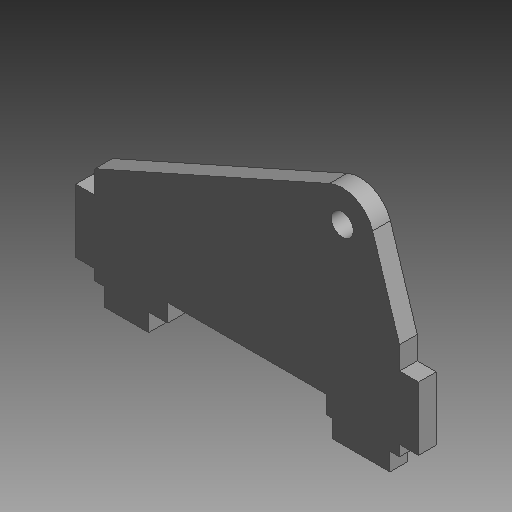
# Autodesk Inventor part: Part15
Saved by Autodesk Inventor 2019.2 (Build 232265000, 265)
## iProperties
Part Number: Part15
Material: Generic
Document SubType Name: Modeling
Designer: richard.girt
Mass: 3.36712 g
Surface Area: 29.1284 cm^2
Volume: 3.36712 cm^3
Density: 1 g/cm^3
Appearance: Default
Author: richard.girt
Autodesk Inventor part; units mm, degrees
note: some values were not read from the file. Chosen so that the rebuilt part matches the saved one: sketch regions of "Extrusion1".
ref_plane "YZ Plane" through (0, 0, 0) normal (1, 0, 0) x (0, 1, 0)
ref_plane "XZ Plane" through (0, 0, 0) normal (0, 1, 0) x (-1, 0, 0)
ref_plane "XY Plane" through (0, 0, 0) normal (0, 0, 1) x (1, 0, 0)
sketch "Sketch1" plane through (0, 0, 0) normal (0, 0, 1) x (1, 0, 0)
  line L0 (24, 7.65) -> (-24, 7.65)
  line L1 (-24, 7.65) -> (-24, -7.65)
  line L2 (-24, -7.65) -> (24, -7.65)
  line L3 (24, -7.65) -> (24, 7.65)
  line L4 (24, 7.65) -> (-24, -7.65) construction
  line L5 (-24, 7.65) -> (24, -7.65) construction
  line L6 (-22.5, -7.65) -> (-15.5, -7.65)
  line L7 (-15.5, -7.65) -> (-15.5, -10.45)
  line L8 (-15.5, -10.45) -> (-22.5, -10.45)
  line L9 (-22.5, -10.45) -> (-22.5, -7.65)
  line L10 (22.5, -7.65) -> (13.5, -7.65)
  line L11 (13.5, -7.65) -> (13.5, -10.45)
  line L12 (13.5, -10.45) -> (22.5, -10.45)
  line L13 (22.5, -10.45) -> (22.5, -7.65)
  line L14 (24, -5.95) -> (27, -5.95)
  line L15 (27, -5.95) -> (27, 4.05)
  line L16 (27, 4.05) -> (24, 4.05)
  line L17 (24, 4.05) -> (24, -5.95)
  line L18 (-24, -5.95) -> (-27, -5.95)
  line L19 (-27, -5.95) -> (-27, 4.05)
  line L20 (-27, 4.05) -> (-24, 4.05)
  line L21 (-24, 4.05) -> (-24, -5.95)
  line L22 (-12.5, -7.65) -> (12.5, -7.65)
  line L23 (12.5, -7.65) -> (12.5, -4.85)
  line L24 (12.5, -4.85) -> (-12.5, -4.85)
  line L25 (-12.5, -4.85) -> (-12.5, -7.65)
  circle A0 centre (15, 19.55) radius 1.75
  arc A1 (19.768, 21.0552) -> (12.9654, 24.1173) centre (15, 19.55) ccw
  line L26 (-24, 7.65) -> (12.9654, 24.1173)
  line L27 (24, 7.65) -> (19.768, 21.0552)
  point P0 (0, 0)
  point P1 (-25.5, -5.95)
  point P2 (25.5, -5.95)
  point P3 (25.5, 4.05)
  point P4 (-25.5, 4.05)
  point P5 (0, -4.85)
  point P6 (0, 0)
  dimension "d0" = 48
  dimension "d1" = 15.3
  dimension "d2" = 3.5
  dimension "d3" = 30
  dimension "d4" = 2.8
  dimension "d5" = 12
  dimension "d6" = 3
  dimension "d7" = 4.5
  dimension "d8" = 10
  dimension "d9" = 25
  dimension "d10" = 7
  dimension "d11" = 9
  dimension "d12" = 4.5
  dimension "d13" = 4.5
  dimension "d14" = 10
  constraints: 56 end point, 12 parallel, 8 midpoint, 6 horizontal, 6 perpendicular, 6 point on line, 2 centre point, 2 equal length, 2 horizontal alignment, 2 point on circle, 2 tangent, 1 coincident, 1 vertical alignment
  measures "d0" distance of L1.end L2.end
  measures "d1" distance of L0.end L1.end
  measures "d2" diameter of A0
  measures "d3" distance from line of L12 A0.centre
  measures "d4" distance of L12.end L10.start
  measures "d5" distance from line of A0.centre L15
  measures "d6" distance of L14.start L14.end
  measures "d7" distance between parallel lines of L14 L12
  measures "d8" distance of L14.end L15.end
  measures "d9" distance of L23.end L24.end
  measures "d10" distance of L7.end L8.end
  measures "d11" distance of L11.end L12.end
  measures "d12" distance between parallel lines of L13 L15
  measures "d13" distance between parallel lines of L19 L9
  measures "d14" diameter of A1
extrude "Extrusion1" add sketch "Sketch1" along normal mid plane 2.8 contours L3 L2 L23 L24 L25 L1 L0 | L0 L26 A1 L27 | L16 L15 L14 L3 | L1 L18 L19 L20 | L13 L12 L11 L2 | L2 L7 L8 L9
body "Solid1"
